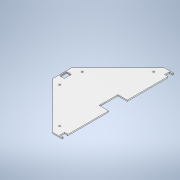
# Autodesk Inventor part: Base 2 Definitiva
Saved by Autodesk Inventor 2021 (Build 250183000, 183)
## iProperties
Created: 2021-04-15
Part Number: Base 2 Definitiva
Material: Plástico ABS
Document SubType Name: Modeling
Designer: Marc
Density: 1.06 g/cm^3
Appearance: Suave - Blanco
Author: Marc
## iProperties of the stored document _3DPrint.ipt
Created: 2021-04-15
Part Number: _3DPrint
Material: Genérico
Document SubType Name: Modeling
Designer: Marc
Density: 1 g/cm^3
Appearance: Valor por defecto
Author: Marc
Autodesk Inventor part; units mm, degrees
ref_plane "YZ Plane" through (0, 0, 0) normal (1, 0, 0) x (0, 1, 0)
ref_plane "XZ Plane" through (0, 0, 0) normal (0, 1, 0) x (-1, 0, 0)
ref_plane "XY Plane" through (0, 0, 0) normal (0, 0, 1) x (1, 0, 0)
sketch "Boceto1" plane through (0, 0, 0) normal (0, 1, 0) x (-1, 0, 0)
  line L0 (0, 145) -> (24.25, 145)
  line L1 (145, 24.25) -> (145, -24.25)
  line L2 (145, 24.25) -> (24.25, 145)
  line L3 (24.25, -145) -> (145, -24.25)
  line L4 (24.25, -145) -> (0, -145)
  circle A0 centre (29.25, -122) radius 2
  circle A1 centre (122, -29.25) radius 2
  circle A2 centre (122, 29.25) radius 2
  circle A3 centre (29.25, 122) radius 2
  line L5 (0, -145) -> (0, 145)
  point P0 (0, 0)
  dimension "d13" = 4
  dimension "d16" = 4
  dimension "d18" = 4
  dimension "d20" = 4
  constraints: 12 end point, 4 centre point, 1 horizontal
  measures "d13" diameter of A0
  measures "d16" diameter of A1
  measures "d18" diameter of A2
  measures "d20" diameter of A3
extrude "Extrusión1" add sketch "Boceto1" along normal blind 3
sketch "Boceto5" plane through (0, 3, 0) normal (0, 1, 0) x (1, 0, 0)
  line L0 (-142, 9) -> (-130, 9)
  line L1 (-130, 9) -> (-130, -9)
  line L2 (-130, -9) -> (-142, -9)
  line L3 (-9, -130) -> (-9, -142)
  line L4 (-9, 130) -> (-9, 142)
  line L5 (-142, 9) -> (-142, -9)
  line L6 (-9, -130) -> (0, -130)
  line L7 (-9, -142) -> (0, -142)
  line L8 (0, -130) -> (0, -142)
  line L9 (0, -145) -> (0, 145) projected
  line L10 (-9, 142) -> (0, 142)
  line L11 (0, 130) -> (0, 142)
  line L12 (-9, 130) -> (0, 130)
  constraints: 24 end point, 3 horizontal, 3 perpendicular, 2 collinear, 2 point on line, 1 parallel
extrude "Extrusión5" cut sketch "Boceto5" against normal blind 3
sketch "Boceto8" plane through (0, 3, 0) normal (0, 1, 0) x (1, 0, 0)
  line L0 (0, 24.25) -> (-24.25, 24.25)
  line L1 (0, -24.25) -> (0, 24.25)
  line L2 (-24.25, 24.25) -> (-24.25, -24.25)
  line L3 (-24.25, -24.25) -> (0, -24.25)
  constraints: 8 end point, 1 horizontal, 1 perpendicular, 1 vertical
extrude "Extrusión8" cut sketch "Boceto8" against normal blind 3
